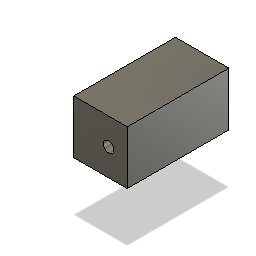
LRF Support Post v4 (Autodesk Fusion 360 design; units mm, degrees)
Autodesk Fusion 360 part; units mm, degrees
sketch "Sketch1" plane through (0, 0, 0) normal (0, 0, 1) x (1, 0, 0)
  line L0 (0, 0) -> (10.16, 0)
  line L1 (10.16, 0) -> (10.16, 10.16)
  line L2 (10.16, 10.16) -> (0, 10.16)
  line L3 (0, 10.16) -> (0, 0)
  circle A0 centre (6.604, 5.08) radius 1.016
  circle A1 centre (-3.81, -4.3942) radius 1.016
  line L4 (7.6211, 0) -> (-0.6691, -8.2902)
  line L5 (7.6211, 0) -> (20.9233, 0) construction
  line L6 (-3.3632, -9.4061) -> (-5.0642, -9.4061)
  line L7 (-8.8742, -5.5961) -> (-8.8742, -1.5782)
  line L8 (-7.7583, 1.1159) -> (0, 8.8742)
  arc A2 (-3.3632, -9.4061) -> (-0.6691, -8.2902) centre (-3.3632, -5.5961) ccw
  arc A3 (-8.8742, -5.5961) -> (-5.0642, -9.4061) centre (-5.0642, -5.5961) ccw
  arc A4 (-7.7583, 1.1159) -> (-8.8742, -1.5782) centre (-5.0642, -1.5782) ccw
  dimension "d1" = 10.16
  dimension "d2" = 10.16
  dimension "d3" = 2.032
  dimension "d4" = 3.556
  dimension "d5" = 5.08
  dimension "d6" = 2.032
  dimension "d7" = 4.3942
  dimension "d8" = 3.81
  dimension "d9" = 135
  dimension "d10" = 135
  dimension "d11" = 3.81
  dimension "d12" = 3.81
  dimension "d13" = 3.81
  constraint horizontal L0
  constraint vertical L1
  constraint horizontal L2
  constraint vertical L3
  constraint coincident L0.start L3.end
  constraint horizontal L5
  constraint coincident L0 L4.start
  constraint parallel L0 L6
  constraint perpendicular L0 L7
  constraint coincident L3 L8.end
  constraint tangent L4 A2
  constraint tangent L6 A2
  constraint tangent L6 A3
  constraint tangent L7 A3
  constraint tangent L7 A4
  constraint tangent L8 A4
  measures "d1" distance of L0.start L0.end
  measures "d2" distance of L0.start L2.end
  measures "d3" diameter of A0
  measures "d4" distance of L1 A0.centre
  measures "d5" distance of L0 A0.centre
  measures "d6" diameter of A1
  measures "d7" distance of L0 A1.centre
  measures "d8" distance of L3 A1.centre
  measures "d9" angle of L4 L5
  measures "d10" angle of L7 L8
  measures "d11" radius of A2
  measures "d12" radius of A3
  measures "d13" radius of A4
extrude "Extrude1" add sketch "Sketch1" along normal blind 19.3294 contours L0 L1 L2 L3
extrude "Extrude2" add sketch "Sketch1" along normal blind 6.604 contours L0 L3 L4 L6 L7 L8 A2 A3 A4
extrude "Extrude3" add sketch "Sketch1" along normal blind 6.604 contours A1
extrude "Extrude4" cut sketch "Sketch1" along normal blind 5.588 contours A1
extrude "Extrude5" add sketch "Sketch1" along normal blind 12.7 contours A0
